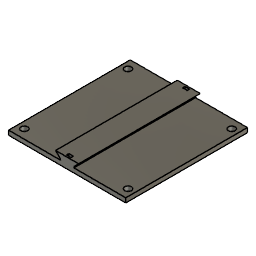
base_bottom (Autodesk Fusion 360 design; units mm, degrees)
part number: 2026-03-16-14-32-38-053
Autodesk Fusion 360 part; units mm, degrees
sketch "Sketch5" plane through (0, 0, 0) normal (0, 0, 1) x (1, 0, 0)
  line L0 (66.04, -66.04) -> (-66.04, -66.04)
  line L1 (-66.04, -66.04) -> (-66.04, 66.04)
  line L2 (-66.04, 66.04) -> (66.04, 66.04)
  line L3 (66.04, 66.04) -> (66.04, -66.04)
  line L4 (66.04, -66.04) -> (-66.04, 66.04) construction
  line L5 (-66.04, -66.04) -> (66.04, 66.04) construction
  constraint horizontal L0
  constraint perpendicular L0 L1
  constraint parallel L0 L2
  constraint parallel L1 L3
  constraint coincident L4 origin
  constraint coincident L5 origin
extrude "Extrude8" add sketch "Sketch5" along normal blind 5.08 makes body 1
sketch "Sketch6" plane through (0, 0, 5.08) normal (0, 0, 1) x (-1, 0, 0)
  line L0 (-66.04, -66.04) -> (66.04, -66.04)
  line L1 (66.04, -66.04) -> (66.04, 66.04)
  line L2 (66.04, 66.04) -> (-66.04, 66.04)
  line L3 (-66.04, 66.04) -> (-66.04, -66.04)
  circle A0 centre (58.42, -58.42) radius 3.81
  circle A1 centre (-58.42, -58.42) radius 3.81
  circle A2 centre (58.42, 58.42) radius 3.81
  circle A3 centre (-58.42, 58.42) radius 3.81
  dimension "d26" = 7.62
  dimension "d27" = 7.62
  dimension "d28" = 7.62
  dimension "d29" = 7.62
  measures "d26" diameter of A0
  measures "d27" diameter of A1
  measures "d28" diameter of A2
  measures "d29" diameter of A3
extrude "Extrude9" cut sketch "Sketch6" against normal blind 15.24 contours A0 | A1 | A2 | A3 bodies 1
sketch "Sketch7" plane through (0, 0, 5.08) normal (0, 0, 1) x (-1, 0, 0)
  circle A0 centre (58.42, -58.42) radius 3.81
  circle A1 centre (-58.42, -58.42) radius 3.81
  circle A2 centre (58.42, 58.42) radius 3.81
  circle A3 centre (-58.42, 58.42) radius 3.81
  line L0 (-66.04, -66.04) -> (66.04, -66.04)
  line L1 (66.04, -66.04) -> (66.04, 66.04)
  line L2 (66.04, 66.04) -> (-66.04, 66.04)
  line L3 (-66.04, 66.04) -> (-66.04, -66.04)
  circle A4 centre (0, 0) radius 62.8904
  dimension "d32" = 125.7808
  constraint coincident A4.centre origin
  measures "d32" diameter of A4
sketch "Sketch8" plane through (0, 0, 0) normal (0, 1, 0) x (1, 0, 0)
  line L0 (-7.62, -7.62) -> (-13.006, -13.0103)
  line L1 (7.62, -7.62) -> (13.0103, -13.006)
  line L2 (13.0103, -13.006) -> (-13.006, -13.0103)
  line L3 (7.62, -7.62) -> (-7.62, -7.62)
  dimension "d35" = 7.62
  dimension "d36" = 7.62
  constraint perpendicular L0 L1
  constraint horizontal L3
  measures "d35" distance of L0.start L0.end
  measures "d36" distance of L1.start L1.end
extrude "Extrude11" add sketch "Sketch8" along normal blind 63.5 and the other way blind 63.5 separate body makes body 2
move_body "Move1" bodies 2 to x (1, 0, 0) y (0, 1, 0) z (0, 0, 1) at (-0.0004, 0, -2.54)
move_body "Move2" bodies 2 to x (1, 0, 0) y (0, 1, 0) z (0, 0, 1) at (0.0004, 0, 2.54)
extrude "Extrude12" add 1 faces at (2.54, -21.1667, 7.62) along direction (0, 0, -1) blind 3.81 separate body on bodies 2 makes body 3
extrude "Extrude13" add 2 faces at (2.5414, 63.5, 11.2121) (2.54, 63.5, 6.35) along direction (0, 1, 0) blind 2.54 separate body on bodies 2 3 makes body 4
extrude "Extrude14" add 2 faces at (2.5414, -63.5, 11.2121) (2.54, -63.5, 6.35) along direction (0, -1, 0) blind 2.54 separate body on bodies 2 3 makes body 5
combine "Combine1" operation add target body 2 tool bodies 4 5 3
move_body "Move3" bodies 2 to x (1, 0, 0) y (0, 1, 0) z (0, 0, 1) at (-0.0001, 0, -0.762)
move_body "Move4" bodies 2 to x (1, 0, 0) y (0, 1, 0) z (0, 0, 1) at (-0.0001, 0, -0.508)
sketch "Sketch9" plane through (0, 0, 5.08) normal (0, 0, 1) x (-1, 0, 0)
  circle A0 centre (58.42, -58.42) radius 3.81
  circle A1 centre (-58.42, -58.42) radius 3.81
  circle A2 centre (58.42, 58.42) radius 3.81
  circle A3 centre (-58.42, 58.42) radius 3.81
  line L0 (-66.04, -66.04) -> (66.04, -66.04)
  line L1 (66.04, -66.04) -> (66.04, 66.04)
  line L2 (66.04, 66.04) -> (-66.04, 66.04)
  line L3 (-66.04, 66.04) -> (-66.04, -66.04)
  line L4 (2.5007, -66.7107) -> (-2.6058, -66.7107)
  line L5 (-2.6058, -66.7107) -> (-2.6058, -64.1707)
  line L6 (-2.6058, -64.1707) -> (2.5007, -64.1707)
  line L7 (2.5007, -64.1707) -> (2.5007, -66.7107)
  line L8 (2.5007, 66.7281) -> (-2.5484, 66.7281)
  line L9 (-2.5484, 66.7281) -> (-2.5484, 64.1881)
  line L10 (-2.5484, 64.1881) -> (2.5007, 64.1881)
  line L11 (2.5007, 64.1881) -> (2.5007, 66.7281)
  constraint horizontal L4
  constraint vertical L5
  constraint horizontal L6
  constraint vertical L7
  constraint horizontal L8
  constraint vertical L9
  constraint horizontal L10
  constraint vertical L11
extrude "Extrude15" add 2 faces at (2.5412, -66.04, 9.9421) (-22.0133, -66.04, 3.3867) along direction (0, -1, 0) blind 2.54 on bodies 1 2 bodies 1 2
extrude "Extrude16" add 2 faces at (-2.5401, 66.04, 1.6933) (2.5412, 66.04, 9.9421) along direction (0, 1, 0) blind 2.54 on bodies 1 bodies 1
extrude "Extrude17" cut sketch "Sketch9" along normal blind 12.7 and the other way blind 10.16 contours L0 L5 L6 L7 | L0 L4 L5 L7 | L2 L8 L9 L11 | L2 L9 L10 L11 bodies 1
